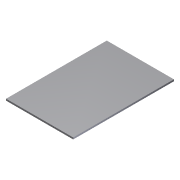
# Autodesk Inventor part: CNC
Saved by Autodesk Inventor 2011 SP1 (Build 150282100, 282)
## iProperties
Created: 2012-11-29
Part Number: CNC
Document SubType Name: Modeling
Designer: arihon
Density: 1 g/cm^3
Author: arihon
Autodesk Inventor part; units mm, degrees
ref_plane "YZ Plane" through (0, 0, 0) normal (1, 0, 0) x (0, 1, 0)
ref_plane "XZ Plane" through (0, 0, 0) normal (0, 1, 0) x (-1, 0, 0)
ref_plane "XY Plane" through (0, 0, 0) normal (0, 0, 1) x (1, 0, 0)
sketch "スケッチ1" plane through (0, 0, 0) normal (0, 0, 1) x (1, 0, 0)
  line L0 (-100, 150) -> (100, 150)
  line L1 (100, 150) -> (100, -150)
  line L2 (100, -150) -> (-100, -150)
  line L3 (-100, -150) -> (-100, 150)
  point P0 (0, 0)
  dimension "d0" = 200
  dimension "d1" = 100
  dimension "d2" = 300
  dimension "d3" = 150
  constraints: 8 end point, 2 parallel, 1 horizontal, 1 perpendicular
  measures "d0" distance of L1.end L2.end
  measures "d1" distance from line of L3 point (0, 0)
  measures "d2" distance of L2.end L0.start
  measures "d3" distance from line of L2 point (0, 0)
extrude "押し出し1" add sketch "スケッチ1" along normal blind 5
equation "\"d1\" = 0.5 * d0"
equation "\"d3\" = 0.5 * d2"
